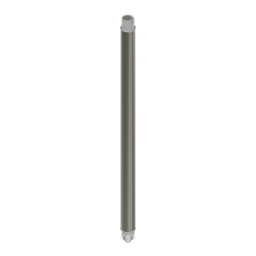
Handle (Autodesk Fusion 360 design; units mm, degrees)
Autodesk Fusion 360 part; units mm, degrees
cylinder "CylinderPrimitive1" add diameter 7.9248 height 142.875 placed x (1, 0, 0) y (0, 1, 0) z (0, 0, 1) at (0, 0, 0)
sketch "Sketch2" plane through (0, 0, 0) normal (0, 0, -1) x (1, 0, 0)
  circle A0 centre (0, 0) radius 3.9624
  circle A1 centre (0, 0) radius 3.175
  dimension "d3" = 6.35
  constraint concentric A0 A1
  measures "d3" diameter of A1
extrude "Extrude1" cut sketch "Sketch2" against normal blind 6.35
thread "Thread1" "ANSI Unified Screw Threads 0.25 1/4-20 UNC 3A" major diameter 6.2484 minor diameter 4.8387 pitch 1.27 angle 60 modelled right hand crest width 0.1965 on face at (3.1592, 0.3161, 4.2333) from (0, 0, 0) to (0, 0, 6.35) crest through (3.1242, 0, -0.3175)
extrude "Extrude2" cut sketch "Sketch2" along normal blind 6.35 from surface at -142.875
thread "Thread2" "ANSI Unified Screw Threads 0.25 1/4-20 UNC 3A" major diameter 6.2484 minor diameter 4.8387 pitch 1.27 angle 60 modelled right hand crest width 0.1965 on face at (3.1592, 0.3161, 138.6417) from (0, 0, 142.875) to (0, 0, 136.525) crest through (3.1242, 0, 143.1925)
